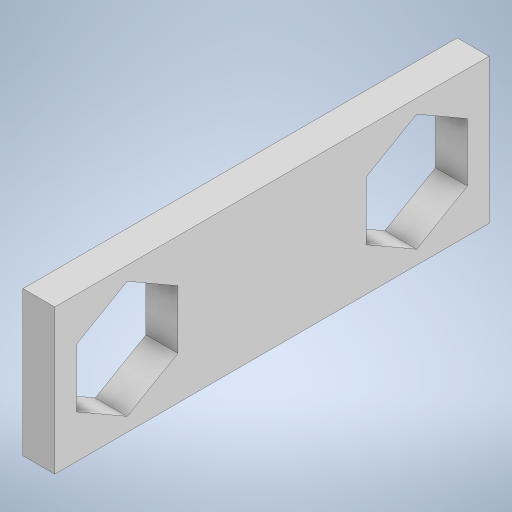
# Autodesk Inventor part: Pengunci sendok - mur
Saved by Autodesk Inventor 2024 (Build 280153000, 153)
## iProperties
Created: 2023-10-30
Part Number: Pengunci sendok - mur
Material: Generic
Document SubType Name: Modeling
Designer: lazy1
Density: 1 g/cm^3
Appearance: Default
Author: lazy1
Autodesk Inventor part; units mm, degrees
ref_plane "YZ Plane" through (0, 0, 0) normal (1, 0, 0) x (0, 1, 0)
ref_plane "XZ Plane" through (0, 0, 0) normal (0, 1, 0) x (-1, 0, 0)
ref_plane "XY Plane" through (0, 0, 0) normal (0, 0, 1) x (1, 0, 0)
sketch "Sketch1" plane through (0, 0, 0) normal (0, 1, 0) x (-1, 0, 0)
  line L0 (-1.1, 15) -> (1.1, 15)
  line L1 (1.1, 15) -> (1.1, -15)
  line L2 (1.1, -15) -> (-1.1, -15)
  line L3 (-1.1, -15) -> (-1.1, 15)
  line L4 (-1.1, 15) -> (1.1, -15) construction
  line L5 (1.1, 15) -> (-1.1, -15) construction
  point P0 (0, 0)
  dimension "d0" = 2.2
  dimension "d1" = 30
  constraints: 12 end point, 2 midpoint, 2 parallel, 1 horizontal, 1 perpendicular
  measures "d0" distance of L1.end L2.end
  measures "d1" distance of L0.end L1.end
extrude "Extrusion1" add sketch "Sketch1" along normal blind 10
sketch "Sketch4" plane through (1.1, 0, 15) normal (1, 0, 0) x (0, 0, -1)
  line L0 (0, 0) -> (0, 10) projected
  line L1 (0, 5) -> (5, 5)
  line L2 (30, 0) -> (30, 10) projected
  line L3 (30, 5) -> (25, 5)
  line L4 (5, 9.0415) -> (8.5, 7.0207)
  line L5 (8.5, 7.0207) -> (8.5, 2.9793)
  line L6 (8.5, 2.9793) -> (5, 0.9585)
  line L7 (5, 0.9585) -> (1.5, 2.9793)
  line L8 (1.5, 2.9793) -> (1.5, 7.0207)
  line L9 (1.5, 7.0207) -> (5, 9.0415)
  line L10 (25, 9.0415) -> (28.5, 7.0207)
  line L11 (28.5, 7.0207) -> (28.5, 2.9793)
  line L12 (28.5, 2.9793) -> (25, 0.9585)
  line L13 (25, 0.9585) -> (21.5, 2.9793)
  line L14 (21.5, 2.9793) -> (21.5, 7.0207)
  line L15 (21.5, 7.0207) -> (25, 9.0415)
  point P0 (15, 0)
  point P1 (28.5, 5)
  point P2 (21.5, 5)
  dimension "d18" = 5
  dimension "d19" = 5
  dimension "d20" = 7
  dimension "d21" = 7
  constraints: 28 end point, 4 midpoint, 2 coincident, 2 horizontal, 26 other
  measures "d18" distance of L1.start L1.end
  measures "d19" distance of L3.start L3.end
  measures "d20" distance between parallel lines of L5 L8
  measures "d21" distance of point (28.5, 5) point (21.5, 5)
extrude "Extrusion3" cut sketch "Sketch4" against normal blind 2.2
body "Solid1"
